IKEA VIHALS (Autodesk Fusion 360 design; units mm, degrees)
Autodesk Fusion 360 part; units mm, degrees
sketch "Sketch1" plane through (0, 0, 0) normal (0, 0, 1) x (1, 0, 0)
  line L0 (-370, 370) -> (370, 370)
  line L1 (370, 370) -> (370, -370)
  line L2 (370, -370) -> (-370, -370)
  line L3 (-370, -370) -> (-370, 370)
  dimension "d1" = 740
  dimension "d2" = 370
  dimension "d3" = 740
  dimension "d4" = 370
  constraint horizontal L0
  constraint vertical L1
  constraint horizontal L2
  constraint vertical L3
  measures "d1" distance of L1 L3
  measures "d2" distance of origin L1
  measures "d3" distance of L0 L2
  measures "d4" distance of origin L0
extrude "Extrude1" add sketch "Sketch1" along normal blind 20
sketch "Sketch3" plane through (0, 0, 0) normal (0, 0, -1) x (1, 0, 0)
  line L0 (370, 370) -> (-370, 370)
  line L1 (-370, 370) -> (-370, -370)
  line L2 (-370, -370) -> (370, -370)
  line L3 (370, -370) -> (370, 370)
  line L4 (360, 365) -> (340, 365)
  line L5 (340, 365) -> (340, 315)
  line L6 (340, 315) -> (360, 315)
  line L7 (360, 315) -> (360, 365)
  line L8 (360, -315) -> (340, -315)
  line L9 (340, -315) -> (340, -365)
  line L10 (340, -365) -> (360, -365)
  line L11 (360, -365) -> (360, -315)
  line L12 (-340, -315) -> (-360, -315)
  line L13 (-360, -315) -> (-360, -365)
  line L14 (-360, -365) -> (-340, -365)
  line L15 (-340, -365) -> (-340, -315)
  line L16 (-340, 365) -> (-360, 365)
  line L17 (-360, 365) -> (-360, 315)
  line L18 (-360, 315) -> (-340, 315)
  line L19 (-340, 315) -> (-340, 365)
  dimension "d7" = 50
  dimension "d8" = 20
  dimension "d9" = 10
  dimension "d10" = 5
  dimension "d11" = 20
  dimension "d12" = 10
  dimension "d13" = 5
  dimension "d14" = 50
  constraint horizontal L4
  constraint vertical L5
  constraint horizontal L6
  constraint vertical L7
  constraint horizontal L8
  constraint vertical L9
  constraint horizontal L10
  constraint vertical L11
  constraint horizontal L12
  constraint vertical L13
  constraint horizontal L14
  constraint vertical L15
  constraint horizontal L16
  constraint vertical L17
  constraint horizontal L18
  constraint vertical L19
  constraint vertical L6.end L8.start
  constraint horizontal L10.end L13.end
  constraint vertical L13.end L16.end
  constraint horizontal L4.start L16.end
  constraint horizontal L5.end L18.end
  constraint vertical L5.end L8.end
  constraint horizontal L8.end L12.start
  constraint vertical L12.start L18.end
  measures "d7" distance of L4 L6
  measures "d8" distance of L5 L7
  measures "d9" distance of L3 L7
  measures "d10" distance of L0 L4
  measures "d11" distance of L17 L19
  measures "d12" distance of L1 L17
  measures "d13" distance of L2 L14
  measures "d14" distance of L12 L14
extrude "Extrude2" add sketch "Sketch3" along normal blind 730 contours L4 L5 L6 L7 | L8 L9 L10 L11 | L12 L13 L14 L15 | L16 L17 L18 L19
sketch "Sketch4" plane through (0, 0, 0) normal (0, 0, -1) x (1, 0, 0)
  line L0 (-340, 315) -> (-360, 315)
  line L1 (-360, 315) -> (-360, 365)
  line L2 (-360, 365) -> (-340, 365)
  line L3 (-340, 365) -> (-340, 315)
  line L4 (360, 315) -> (340, 315)
  line L5 (340, 315) -> (340, 365)
  line L6 (340, 365) -> (360, 365)
  line L7 (360, 365) -> (360, 315)
  line L8 (-340, -365) -> (-360, -365)
  line L9 (-360, -365) -> (-360, -315)
  line L10 (-360, -315) -> (-340, -315)
  line L11 (-340, -315) -> (-340, -365)
  line L12 (360, -365) -> (340, -365)
  line L13 (340, -365) -> (340, -315)
  line L14 (340, -315) -> (360, -315)
  line L15 (360, -315) -> (360, -365)
  line L16 (370, 370) -> (-370, 370)
  line L17 (-370, 370) -> (-370, -370)
  line L18 (-370, -370) -> (370, -370)
  line L19 (370, -370) -> (370, 370)
  line L20 (-340, 334) -> (340, 334)
  line L21 (340, 334) -> (340, 319)
  line L22 (340, 319) -> (-340, 319)
  line L23 (-340, 319) -> (-340, 334)
  line L24 (-340, -319) -> (340, -319)
  line L25 (340, -319) -> (340, -334)
  line L26 (340, -334) -> (-340, -334)
  line L27 (-340, -334) -> (-340, -319)
  line L28 (344, 315) -> (359, 315)
  line L29 (359, 315) -> (359, -315)
  line L30 (359, -315) -> (344, -315)
  line L31 (344, -315) -> (344, 315)
  line L32 (-359, 315) -> (-344, 315)
  line L33 (-344, 315) -> (-344, -315)
  line L34 (-344, -315) -> (-359, -315)
  line L35 (-359, -315) -> (-359, 315)
  dimension "d17" = 15
  dimension "d18" = 15
  dimension "d19" = 15
  dimension "d20" = 15
  dimension "d21" = 630
  dimension "d22" = 680
  dimension "d23" = 55
  dimension "d24" = 30
  dimension "d25" = 11
  dimension "d26" = 11
  dimension "d27" = 4
  dimension "d28" = 4
  constraint horizontal L20
  constraint vertical L21
  constraint horizontal L22
  constraint vertical L23
  constraint horizontal L24
  constraint vertical L25
  constraint horizontal L26
  constraint vertical L27
  constraint horizontal L28
  constraint vertical L29
  constraint horizontal L30
  constraint vertical L31
  constraint horizontal L32
  constraint vertical L33
  constraint horizontal L34
  constraint vertical L35
  constraint horizontal L28.start L32.end
  constraint vertical L22.end L24.start
  constraint vertical L21.end L24.end
  constraint horizontal L30.end L33.end
  measures "d17" distance of L33 L35
  measures "d18" distance of L20 L22
  measures "d19" distance of L24 L26
  measures "d20" distance of L29 L31
  measures "d21" distance of L32 L34
  measures "d22" distance of L25 L27
  measures "d23" distance of L18 L34
  measures "d24" distance of L17 L27
  measures "d25" distance of L17 L35
  measures "d26" distance of L19 L29
  measures "d27" distance of L22 L32
  measures "d28" distance of L14 L24
extrude "Extrude3" add sketch "Sketch4" along normal blind 40 contours L0 L10 L32 L33 L34 L35 | L3 L5 L20 L21 L22 L23 | L11 L13 L24 L25 L26 L27 | L4 L14 L28 L29 L30 L31
sketch "Sketch5" plane through (0, 0, 0) normal (0, 0, -1) x (1, 0, 0)
  line L0 (344, -315) -> (344, 315)
  line L1 (344, 315) -> (340, 315)
  line L2 (340, 315) -> (340, 319)
  line L3 (340, 319) -> (-340, 319)
  line L4 (-340, 319) -> (-340, 315)
  line L5 (-340, 315) -> (-344, 315)
  line L6 (-344, 315) -> (-344, -315)
  line L7 (-344, -315) -> (-340, -315)
  line L8 (-340, -315) -> (-340, -319)
  line L9 (-340, -319) -> (340, -319)
  line L10 (340, -319) -> (340, -315)
  line L11 (340, -315) -> (344, -315)
  line L12 (344, -295) -> (320, -319)
  line L13 (344, -280) -> (305, -319)
  line L14 (-320, -319) -> (-344, -295)
  line L15 (-344, -280) -> (-305, -319)
  line L16 (344, 295) -> (320, 319)
  line L17 (344, 280) -> (305, 319)
  line L18 (-320, 319) -> (-344, 295)
  line L19 (-305, 319) -> (-344, 280)
  dimension "d31" = 45
  dimension "d32" = 45
  dimension "d33" = 20
  dimension "d34" = 15
  dimension "d35" = 45
  dimension "d36" = 45
  dimension "d37" = 15
  dimension "d38" = 20
  dimension "d39" = 45
  dimension "d40" = 45
  dimension "d41" = 20
  dimension "d42" = 15
  dimension "d43" = 45
  dimension "d44" = 45
  dimension "d45" = 20
  dimension "d46" = 15
  constraint coincident L0 L12.start
  constraint coincident L9 L12.end
  constraint coincident L0 L13.start
  constraint coincident L9 L13.end
  constraint coincident L9 L14.start
  constraint coincident L6 L14.end
  constraint coincident L6 L15.start
  constraint coincident L9 L15.end
  constraint coincident L0 L16.start
  constraint coincident L3 L16.end
  constraint coincident L0 L17.start
  constraint coincident L3 L17.end
  constraint coincident L3 L18.start
  constraint coincident L6 L18.end
  constraint coincident L3 L19.start
  constraint coincident L6 L19.end
  measures "d31" angle of L0 L12
  measures "d32" angle of L0 L13
  measures "d33" distance of L0.start L12.start
  measures "d34" distance of L12.start L13.start
  measures "d35" angle of L6 L14
  measures "d36" angle of L6 L15
  measures "d37" distance of L14.end L15.start
  measures "d38" distance of L6.end L14.end
  measures "d39" angle of L0 L16
  measures "d40" angle of L0 L17
  measures "d41" distance of L0.end L16.start
  measures "d42" distance of L16.start L17.start
  measures "d43" angle of L3 L19
  measures "d44" angle of L3 L18
  measures "d45" distance of L5.end L18.end
  measures "d46" distance of L18.end L19.end
extrude "Extrude4" add sketch "Sketch5" along normal blind 40 contours L0 L9 L12 L13 | L0 L3 L16 L17 | L6 L9 L14 L15 | L3 L6 L18 L19
equation "d2 = ( 740 / 2 ) * 1 mm"
equation "d4 = ( 740 / 2 ) * 1 mm"
equation "d23 = ( ( 740 - 630 ) / 2 ) * 1 mm"
equation "d24 = ( ( 740 - 680 ) / 2 ) * 1 mm"
